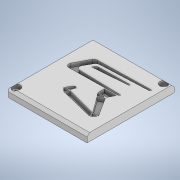
# Autodesk Inventor part: logo_do_obudowy
Saved by Autodesk Inventor 2022 (Build 260153000, 153)
## iProperties
Created: 2022-10-25
Part Number: logo_do_obudowy
Material: Generic
Document SubType Name: Modeling
Designer: Kamil
Density: 1 g/cm^3
Appearance: Default
Author: Kamil
Autodesk Inventor part; units mm, degrees
ref_plane "YZ Plane" through (0, 0, 0) normal (1, 0, 0) x (0, 1, 0)
ref_plane "XZ Plane" through (0, 0, 0) normal (0, 1, 0) x (-1, 0, 0)
ref_plane "XY Plane" through (0, 0, 0) normal (0, 0, 1) x (1, 0, 0)
sketch "Sketch1" plane through (0, 0, 0) normal (0, 1, 0) x (-1, 0, 0)
  line L0 (17.0032, 34.9779) -> (23.3361, 34.9779)
  arc A0 (23.5361, 34.7779) -> (23.3361, 34.9779) centre (23.3361, 34.7779) ccw
  line L1 (23.5361, 34.7779) -> (23.5361, 30.4736)
  arc A1 (23.3402, 30.2737) -> (23.5361, 30.4736) centre (23.3361, 30.4736) ccw
  line L2 (23.3402, 30.2737) -> (14.6312, 30.0942)
  arc A2 (14.4504, 30.3878) -> (14.6312, 30.0942) centre (14.6271, 30.2941) ccw
  line L3 (14.4504, 30.3878) -> (16.8265, 34.8716)
  arc A3 (17.0032, 34.9779) -> (16.8265, 34.8716) centre (17.0032, 34.7779) ccw
  line L4 (11.4862, 54.1871) -> (36.5401, 47.9784)
  arc A4 (36.6796, 47.7151) -> (36.5401, 47.9784) centre (36.492, 47.7843) ccw
  line L5 (36.6796, 47.7151) -> (35.6192, 44.8386)
  arc A5 (35.3802, 44.7145) -> (35.6192, 44.8386) centre (35.4315, 44.9078) ccw
  line L6 (35.3802, 44.7145) -> (12.7355, 50.7268)
  arc A6 (12.6037, 50.8398) -> (12.7355, 50.7268) centre (12.7869, 50.9201) ccw
  line L7 (12.6037, 50.8398) -> (11.255, 53.9126)
  arc A7 (11.4862, 54.1871) -> (11.255, 53.9126) centre (11.4381, 53.9929) ccw
  line L8 (39.8584, 45.0104) -> (36.5274, 44.6997)
  arc A8 (36.3265, 44.9811) -> (36.5274, 44.6997) centre (36.5088, 44.8988) ccw
  line L9 (36.3265, 44.9811) -> (37.4459, 47.4633)
  arc A9 (37.7683, 47.5238) -> (37.4459, 47.4633) centre (37.6282, 47.3811) ccw
  line L10 (37.7683, 47.5238) -> (39.98, 45.3522)
  arc A10 (39.8584, 45.0104) -> (39.98, 45.3522) centre (39.8398, 45.2095) ccw
  line L11 (21.7451, 37.7147) -> (23.0956, 35.9715)
  arc A11 (22.9375, 35.649) -> (23.0956, 35.9715) centre (22.9375, 35.849) ccw
  line L12 (22.9375, 35.649) -> (18.4582, 35.649)
  arc A12 (18.3608, 36.0237) -> (18.4582, 35.649) centre (18.4582, 35.849) ccw
  line L13 (18.3608, 36.0237) -> (21.4896, 37.7669)
  arc A13 (21.7451, 37.7147) -> (21.4896, 37.7669) centre (21.587, 37.5922) ccw
  arc A14 (40.0803, 18.0118) -> (42.2272, 19.1869) centre (40.0302, 20.6522) ccw
  line L14 (40.0803, 18.0118) -> (16.2631, 17.5595)
  arc A15 (16.1729, 17.7063) -> (16.2631, 17.5595) centre (16.2612, 17.6595) ccw
  line L15 (16.1729, 17.7063) -> (16.5854, 18.4847)
  arc A16 (16.6657, 18.5376) -> (16.5854, 18.4847) centre (16.6737, 18.4379) ccw
  line L16 (16.6657, 18.5376) -> (42.8686, 20.645)
  line L17 (42.8686, 20.645) -> (43.0978, 20.4922)
  line L18 (43.0978, 20.4922) -> (42.2272, 19.1869)
  line L19 (8.0984, 51.7664) -> (10.3047, 54.0133)
  arc A17 (10.6328, 53.9484) -> (10.3047, 54.0133) centre (10.4474, 53.8732) ccw
  line L20 (10.6328, 53.9484) -> (11.6185, 51.5186)
  arc A18 (11.4217, 51.2437) -> (11.6185, 51.5186) centre (11.4332, 51.4434) ccw
  line L21 (11.4217, 51.2437) -> (8.2297, 51.4266)
  arc A19 (8.0984, 51.7664) -> (8.2297, 51.4266) centre (8.2411, 51.6263) ccw
  line L22 (39.5708, 43.975) -> (36.8282, 39.8589)
  arc A20 (36.5926, 39.7821) -> (36.8282, 39.8589) centre (36.6617, 39.9698) ccw
  line L23 (36.5926, 39.7821) -> (35.0574, 40.3481)
  arc A21 (34.9389, 40.6049) -> (35.0574, 40.3481) centre (35.1266, 40.5358) ccw
  line L24 (34.9389, 40.6049) -> (36.1416, 43.8672)
  arc A22 (36.3106, 43.9972) -> (36.1416, 43.8672) centre (36.3293, 43.798) ccw
  line L25 (36.3106, 43.9972) -> (39.3857, 44.285)
  arc A23 (39.5708, 43.975) -> (39.3857, 44.285) centre (39.4044, 44.0859) ccw
  line L26 (12.3567, 50.5223) -> (20.9275, 38.605)
  arc A24 (20.8625, 38.3135) -> (20.9275, 38.605) centre (20.7651, 38.4882) ccw
  line L27 (20.8625, 38.3135) -> (17.0472, 36.1879)
  arc A25 (16.7814, 36.2548) -> (17.0472, 36.1879) centre (16.9499, 36.3626) ccw
  line L28 (16.7814, 36.2548) -> (7.6775, 50.4817)
  arc A26 (7.8545, 50.7893) -> (7.6775, 50.4817) centre (7.846, 50.5895) ccw
  line L29 (7.8545, 50.7893) -> (12.2028, 50.6053)
  arc A27 (12.3567, 50.5223) -> (12.2028, 50.6053) centre (12.1943, 50.4055) ccw
  arc A28 (45.6629, 13.764) -> (47.9412, 15.166) centre (45.6087, 16.4042) ccw
  line L30 (45.6629, 13.764) -> (4.4501, 12.9186)
  arc A29 (4.3597, 13.0655) -> (4.4501, 12.9186) centre (4.448, 13.0186) ccw
  line L31 (4.3597, 13.0655) -> (4.9465, 14.171)
  arc A30 (5.0303, 14.224) -> (4.9465, 14.171) centre (5.0349, 14.1241) ccw
  line L32 (5.0303, 14.224) -> (41.6378, 15.9024)
  arc A31 (41.6378, 15.9024) -> (44.3506, 17.5585) centre (41.4866, 19.1999) ccw
  line L33 (44.3506, 17.5585) -> (47.7058, 23.4127)
  arc A32 (47.7058, 23.4127) -> (45.4763, 27.3659) centre (45.4146, 24.7258) ccw
  line L34 (45.4763, 27.3659) -> (13.094, 28.122)
  line L35 (13.094, 28.122) -> (13.8544, 29.2632)
  line L36 (13.8544, 29.2632) -> (51.3221, 29.8907)
  arc A33 (53.6988, 26.012) -> (51.3221, 29.8907) centre (51.3663, 27.2502) ccw
  line L37 (53.6988, 26.012) -> (47.9412, 15.166)
  line L38 (0, 0) -> (62.6, 0)
  line L39 (62.6, 0) -> (62.6, 67.2)
  line L40 (62.6, 67.2) -> (0, 67.2)
  line L41 (0, 67.2) -> (0, 0)
  line L42 (0, 0) -> (4, 0)
  line L43 (4, 0) -> (4, 4)
  line L44 (4, 4) -> (0, 4)
  line L45 (0, 4) -> (0, 0)
  line L46 (62.6, 67.2) -> (58.6, 67.2)
  line L47 (58.6, 67.2) -> (58.6, 63.2)
  line L48 (58.6, 63.2) -> (62.6, 63.2)
  line L49 (62.6, 63.2) -> (62.6, 67.2)
  circle A34 centre (4, 4) radius 1.5
  circle A35 centre (58.6, 63.2) radius 1.5
  dimension "d0" = 4
  dimension "d1" = 4
  dimension "d2" = 4
  dimension "d3" = 4
  dimension "d4" = 3
  dimension "d5" = 3
  constraints: 100 end point, 68 point on circle, 36 centre point, 4 parallel, 2 coincident, 2 horizontal, 2 perpendicular, 1 vertical
  measures "d0" distance of L44.end L43.end
  measures "d1" distance of L43.end L42.end
  measures "d2" distance of L48.end L47.end
  measures "d3" distance of L47.end L46.end
  measures "d4" diameter of A34
  measures "d5" diameter of A35
extrude "Extrusion1" add sketch "Sketch1" along normal blind 6 contours L41 L44 A34 L43 L38 | L43 A34 L44 L41 L40 L47 A35 L48 L39 L38 | L48 A35 L47 L40 L39
extrude "Extrusion2" add sketch "Sketch1" along normal blind 3 contours L0 A0 L1 A1 L2 A2 L3 A3 | L4 A4 L5 A5 L6 A6 L7 A7 | L8 A8 L9 A9 L10 A10 | L11 A11 L12 A12 L13 A13 | L14 A15 L15 A16 L16 L17 L18 A14 | L19 A17 L20 A18 L21 A19 | L22 A20 L23 A21 L24 A22 L25 A23 | L26 A24 L27 A25 L28 A26 L29 A27 | L30 A29 L31 A30 L32 A31 L33 A32 L34 L35 L36 A33 L37 A28
sketch "Sketch2" plane through (0, 6, 0) normal (0, 1, 0) x (1, 0, 0)
  line L0 (-62.6, 0) -> (-62.6, -67.2) projected
  line L1 (-62.6, -67.2) -> (0, -67.2) projected
  line L2 (0, -67.2) -> (0, 0) projected
  line L3 (0, 0) -> (-62.6, 0) projected
  circle A0 centre (-4, -4) radius 1.5 projected
  circle A1 centre (-58.6, -63.2) radius 1.5 projected
  line L4 (-36.3106, -43.9972) -> (-39.3857, -44.285) projected
  arc A2 (-39.5708, -43.975) -> (-39.3857, -44.285) centre (-39.4044, -44.0859) ccw projected
  line L5 (-39.5708, -43.975) -> (-36.8282, -39.8589) projected
  arc A3 (-36.5926, -39.7821) -> (-36.8282, -39.8589) centre (-36.6617, -39.9698) ccw projected
  line L6 (-36.5926, -39.7821) -> (-35.0574, -40.3481) projected
  arc A4 (-34.9389, -40.6049) -> (-35.0574, -40.3481) centre (-35.1266, -40.5358) ccw projected
  line L7 (-34.9389, -40.6049) -> (-36.1416, -43.8672) projected
  arc A5 (-36.3106, -43.9972) -> (-36.1416, -43.8672) centre (-36.3293, -43.798) ccw projected
  line L8 (-39.8584, -45.0104) -> (-36.5274, -44.6997) projected
  arc A6 (-36.3265, -44.9811) -> (-36.5274, -44.6997) centre (-36.5088, -44.8988) ccw projected
  line L9 (-36.3265, -44.9811) -> (-37.4459, -47.4633) projected
  arc A7 (-37.7683, -47.5238) -> (-37.4459, -47.4633) centre (-37.6282, -47.3811) ccw projected
  line L10 (-37.7683, -47.5238) -> (-39.98, -45.3522) projected
  arc A8 (-39.8584, -45.0104) -> (-39.98, -45.3522) centre (-39.8398, -45.2095) ccw projected
  line L11 (-42.8686, -20.645) -> (-43.0978, -20.4922) projected
  line L12 (-43.0978, -20.4922) -> (-42.2272, -19.1869) projected
  arc A9 (-40.0803, -18.0118) -> (-42.2272, -19.1869) centre (-40.0302, -20.6522) ccw projected
  line L13 (-40.0803, -18.0118) -> (-16.2631, -17.5595) projected
  arc A10 (-16.1729, -17.7063) -> (-16.2631, -17.5595) centre (-16.2612, -17.6595) ccw projected
  line L14 (-16.1729, -17.7063) -> (-16.5854, -18.4847) projected
  arc A11 (-16.6657, -18.5376) -> (-16.5854, -18.4847) centre (-16.6737, -18.4379) ccw projected
  line L15 (-16.6657, -18.5376) -> (-42.8686, -20.645) projected
  line L16 (-16.7814, -36.2548) -> (-7.6775, -50.4817) projected
  arc A12 (-7.8545, -50.7893) -> (-7.6775, -50.4817) centre (-7.846, -50.5895) ccw projected
  line L17 (-7.8545, -50.7893) -> (-12.2028, -50.6053) projected
  arc A13 (-12.3567, -50.5223) -> (-12.2028, -50.6053) centre (-12.1943, -50.4055) ccw projected
  line L18 (-12.3567, -50.5223) -> (-20.9275, -38.605) projected
  arc A14 (-20.8625, -38.3135) -> (-20.9275, -38.605) centre (-20.7651, -38.4882) ccw projected
  line L19 (-20.8625, -38.3135) -> (-17.0472, -36.1879) projected
  arc A15 (-16.7814, -36.2548) -> (-17.0472, -36.1879) centre (-16.9499, -36.3626) ccw projected
  line L20 (-8.0984, -51.7664) -> (-10.3047, -54.0133) projected
  arc A16 (-10.6328, -53.9484) -> (-10.3047, -54.0133) centre (-10.4474, -53.8732) ccw projected
  line L21 (-10.6328, -53.9484) -> (-11.6185, -51.5186) projected
  arc A17 (-11.4217, -51.2437) -> (-11.6185, -51.5186) centre (-11.4332, -51.4434) ccw projected
  line L22 (-11.4217, -51.2437) -> (-8.2297, -51.4266) projected
  arc A18 (-8.0984, -51.7664) -> (-8.2297, -51.4266) centre (-8.2411, -51.6263) ccw projected
  line L23 (-11.4862, -54.1871) -> (-36.5401, -47.9784) projected
  arc A19 (-36.6796, -47.7151) -> (-36.5401, -47.9784) centre (-36.492, -47.7843) ccw projected
  line L24 (-36.6796, -47.7151) -> (-35.6192, -44.8386) projected
  arc A20 (-35.3802, -44.7145) -> (-35.6192, -44.8386) centre (-35.4315, -44.9078) ccw projected
  line L25 (-35.3802, -44.7145) -> (-12.7355, -50.7268) projected
  arc A21 (-12.6037, -50.8398) -> (-12.7355, -50.7268) centre (-12.7869, -50.9201) ccw projected
  line L26 (-12.6037, -50.8398) -> (-11.255, -53.9126) projected
  arc A22 (-11.4862, -54.1871) -> (-11.255, -53.9126) centre (-11.4381, -53.9929) ccw projected
  line L27 (-23.3402, -30.2737) -> (-14.6312, -30.0942) projected
  arc A23 (-14.4504, -30.3878) -> (-14.6312, -30.0942) centre (-14.6271, -30.2941) ccw projected
  line L28 (-14.4504, -30.3878) -> (-16.8265, -34.8716) projected
  arc A24 (-17.0032, -34.9779) -> (-16.8265, -34.8716) centre (-17.0032, -34.7779) ccw projected
  line L29 (-17.0032, -34.9779) -> (-23.3361, -34.9779) projected
  arc A25 (-23.5361, -34.7779) -> (-23.3361, -34.9779) centre (-23.3361, -34.7779) ccw projected
  line L30 (-23.5361, -34.7779) -> (-23.5361, -30.4736) projected
  arc A26 (-23.3402, -30.2737) -> (-23.5361, -30.4736) centre (-23.3361, -30.4736) ccw projected
  line L31 (-5.0303, -14.224) -> (-41.6378, -15.9024) projected
  arc A27 (-41.6378, -15.9024) -> (-44.3506, -17.5585) centre (-41.4866, -19.1999) ccw projected
  line L32 (-44.3506, -17.5585) -> (-47.7058, -23.4127) projected
  arc A28 (-47.7058, -23.4127) -> (-45.4763, -27.3659) centre (-45.4146, -24.7258) ccw projected
  line L33 (-45.4763, -27.3659) -> (-13.094, -28.122) projected
  line L34 (-13.094, -28.122) -> (-13.8544, -29.2632) projected
  line L35 (-13.8544, -29.2632) -> (-51.3221, -29.8907) projected
  arc A29 (-53.6988, -26.012) -> (-51.3221, -29.8907) centre (-51.3663, -27.2502) ccw projected
  line L36 (-53.6988, -26.012) -> (-47.9412, -15.166) projected
  arc A30 (-45.6629, -13.764) -> (-47.9412, -15.166) centre (-45.6087, -16.4042) ccw projected
  line L37 (-45.6629, -13.764) -> (-4.4501, -12.9186) projected
  arc A31 (-4.3597, -13.0655) -> (-4.4501, -12.9186) centre (-4.448, -13.0186) ccw projected
  line L38 (-4.3597, -13.0655) -> (-4.9465, -14.171) projected
  arc A32 (-5.0303, -14.224) -> (-4.9465, -14.171) centre (-5.0349, -14.1241) ccw projected
  line L39 (-21.7451, -37.7147) -> (-23.0956, -35.9715) projected
  arc A33 (-22.9375, -35.649) -> (-23.0956, -35.9715) centre (-22.9375, -35.849) ccw projected
  line L40 (-22.9375, -35.649) -> (-18.4582, -35.649) projected
  arc A34 (-18.3608, -36.0237) -> (-18.4582, -35.649) centre (-18.4582, -35.849) ccw projected
  line L41 (-18.3608, -36.0237) -> (-21.4896, -37.7669) projected
  arc A35 (-21.7451, -37.7147) -> (-21.4896, -37.7669) centre (-21.587, -37.5922) ccw projected
  circle A36 centre (-4, -4) radius 1.5 projected
  circle A37 centre (-4, -4) radius 3
  circle A38 centre (-58.6, -63.1208) radius 3
  dimension "d10" = 6
  dimension "d11" = 6
  constraints: 2 centre point, 1 coincident
  measures "d10" diameter of A37
  measures "d11" diameter of A38
extrude "Extrusion3" cut sketch "Sketch2" against normal blind 3 contours A37 | A38
chamfer "Chamfer1" distance 2 angle 45 2 edges at (-62.6, 3, 0) (-62.6, 3, 67.2)
chamfer "Chamfer2" distance 2 angle 45 3 edges at (-62.6, 6, 33.6) (-30.3, 6, 0) (-30.3, 6, 67.2)
body "Solid1"
